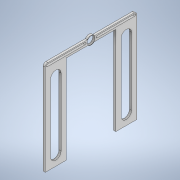
# Autodesk Inventor part: Monitor Part ReDes
Saved by Autodesk Inventor 2020.2 (Build 242310000, 310)
## iProperties
Created: 2020-05-07
Part Number: Monitor Part ReDes
Material: Generic
Document SubType Name: Modeling
Designer: Amaan Khalid
Density: 1 g/cm^3
Appearance: Default
Author: Amaan Khalid
Autodesk Inventor part; units mm, degrees
ref_plane "YZ Plane" through (0, 0, 0) normal (1, 0, 0) x (0, 1, 0)
ref_plane "XZ Plane" through (0, 0, 0) normal (0, 1, 0) x (-1, 0, 0)
ref_plane "XY Plane" through (0, 0, 0) normal (0, 0, 1) x (1, 0, 0)
sketch "Sketch1" plane through (0, 0, 0) normal (1, 0, 0) x (0, 1, 0)
  circle A0 centre (30.6474, 53.9552) radius 5.08
  line L0 (33.2311, 49.5813) -> (33.2311, 1.9563)
  line L1 (33.2311, 58.3291) -> (33.2311, 105.9541)
  line L2 (30.0561, 109.1291) -> (27.0711, 109.1291)
  arc A1 (33.2311, 105.9541) -> (30.0561, 109.1291) centre (30.0561, 105.9541) ccw
  line L3 (30.0561, -1.2187) -> (27.0711, -1.2187)
  arc A2 (30.0561, -1.2187) -> (33.2311, 1.9563) centre (30.0561, 1.9563) ccw
  line L4 (27.0711, 109.1291) -> (27.0711, 57.5631)
  line L5 (27.0711, -1.2187) -> (27.0711, 50.3474)
  line L6 (27.0711, 109.1291) -> (27.0711, 83.7291)
  line L7 (27.0711, 109.1291) -> (-79.6089, 109.1291)
  line L8 (-79.6089, 109.1291) -> (-79.6089, 83.7291)
  line L9 (-79.6089, 83.7291) -> (27.0711, 83.7291)
  line L10 (27.0711, -1.2187) -> (-79.6089, -1.2187)
  line L11 (-79.6089, -1.2187) -> (-79.6089, 24.1813)
  line L12 (27.0711, -1.2187) -> (27.0711, 24.1813)
  line L13 (27.0711, 24.1813) -> (-79.6089, 24.1813)
  circle A3 centre (30.6474, 53.9552) radius 4.7025
  point P0 (33.2311, -1.2187)
  point P1 (33.2311, 109.1291)
  dimension "d3" = 50.8
  dimension "d4" = 50.8
  dimension "d5" = 6.16
  dimension "d6" = 3.175
  dimension "d7" = 3.175
  dimension "d8" = 25.4
  dimension "d9" = 106.68
  dimension "d10" = 106.68
  dimension "d11" = 25.4
  dimension "d13" = 25.4
  constraints: 28 end point, 8 point on circle, 6 point on line, 4 centre point, 4 horizontal, 4 tangent, 3 perpendicular, 3 vertical, 1 coincident
  measures "d3" distance of L0.start point (33.231, -1.219)
  measures "d4" distance of L1.start point (33.231, 109.129)
  measures "d5" distance of point (33.231, 109.129) L2.end
  measures "d6" radius of A1
  measures "d7" radius of A2
  measures "d8" distance of L2.end L6.end
  measures "d9" distance of L2.end L7.end
  measures "d10" distance of L3.end L10.end
  measures "d11" distance of L10.end L11.end
  measures "d13" distance of L3.end L12.end
extrude "Extrusion1" add sketch "Sketch1" along normal blind 2.54 contours A0 | A0 L4 L2 A1 L1 | L0 A2 L3 L5 A0
sketch "Sketch2" plane through (2.54, 0, 0) normal (1, 0, 0) x (0, 0, -1)
  line L0 (-109.1291, 27.0711) -> (-57.5631, 27.0711) projected
  line L1 (-109.1291, 27.0711) -> (-109.1291, -79.6089)
  line L2 (-109.1291, -79.6089) -> (-83.7291, -79.6089)
  line L3 (-83.7291, -79.6089) -> (-83.7291, 27.0711)
  line L4 (-109.1291, 27.0711) -> (-83.7291, 27.0711)
  line L5 (1.2187, 27.0711) -> (1.2187, 30.0561) projected
  line L6 (1.2187, 27.0711) -> (1.2187, -79.6089)
  line L7 (1.2187, -79.6089) -> (-24.1813, -79.6089)
  line L8 (-24.1813, -79.6089) -> (-24.1813, 27.0711)
  line L9 (-50.3474, 27.0711) -> (1.2187, 27.0711) projected
  point P0 (0, 0)
  dimension "d16" = 106.68
  dimension "d17" = 25.4
  dimension "d18" = 106.68
  dimension "d19" = 25.4
  constraints: 14 end point, 3 perpendicular, 2 point on line, 2 vertical, 1 collinear, 1 horizontal
  measures "d16" distance of L0.start L1.end
  measures "d17" distance of L1.end L2.end
  measures "d18" distance of L5.start L6.end
  measures "d19" distance of L6.end L7.end
extrude "Extrusion2" add sketch "Sketch2" against normal up to surface (2.54 mm away)
sketch "Sketch3" plane through (2.54, 0, 0) normal (1, 0, 0) x (0, 0, -1)
  line L0 (-83.7291, -79.6089) -> (-83.7291, 27.0711) projected
  line L1 (-58.3291, 33.2311) -> (-105.9541, 33.2311) projected
  line L2 (-109.1291, 30.0561) -> (-109.1291, -79.6089) projected
  line L3 (-109.1291, -79.6089) -> (-83.7291, -79.6089) projected
  line L4 (-96.4291, 20.7211) -> (-96.4291, 20.7211)
  line L5 (-90.0791, 14.3711) -> (-90.0791, -66.9089)
  line L6 (-96.4291, -73.2589) -> (-96.4291, -73.2589)
  line L7 (-102.7791, -66.9089) -> (-102.7791, 14.3711)
  arc A0 (-96.4291, 20.7211) -> (-102.7791, 14.3711) centre (-96.4291, 14.3711) ccw
  arc A1 (-90.0791, 14.3711) -> (-96.4291, 20.7211) centre (-96.4291, 14.3711) ccw
  arc A2 (-102.7791, -66.9089) -> (-96.4291, -73.2589) centre (-96.4291, -66.9089) ccw
  arc A3 (-96.4291, -73.2589) -> (-90.0791, -66.9089) centre (-96.4291, -66.9089) ccw
  line L8 (-11.4813, 20.7211) -> (-11.4813, 20.7211)
  line L9 (-17.8313, 14.3711) -> (-17.8313, -66.9089)
  line L10 (-11.4813, -73.2589) -> (-11.4813, -73.2589)
  line L11 (-5.1313, -66.9089) -> (-5.1313, 14.3711)
  line L12 (-24.1813, -79.6089) -> (1.2187, -79.6089) projected
  line L13 (-50.3474, 27.0711) -> (-24.1813, 27.0711) projected
  line L14 (1.2187, -79.6089) -> (1.2187, 30.0561) projected
  line L15 (-24.1813, 27.0711) -> (-24.1813, -79.6089) projected
  arc A4 (-11.4813, 20.7211) -> (-17.8313, 14.3711) centre (-11.4813, 14.3711) ccw
  arc A5 (-5.1313, 14.3711) -> (-11.4813, 20.7211) centre (-11.4813, 14.3711) ccw
  arc A6 (-17.8313, -66.9089) -> (-11.4813, -73.2589) centre (-11.4813, -66.9089) ccw
  arc A7 (-11.4813, -73.2589) -> (-5.1313, -66.9089) centre (-11.4813, -66.9089) ccw
  circle A8 centre (-53.9552, 30.6474) radius 4.7025 projected
  line L16 (-58.6577, 30.6474) -> (-61.1977, 30.6474)
  arc A9 (-61.1977, 29.3774) -> (-61.1977, 31.9174) centre (-61.1977, 30.6474) ccw
  line L17 (-109.1291, 30.6474) -> (-106.5891, 30.6474)
  arc A10 (-106.5891, 31.9174) -> (-106.5891, 29.3774) centre (-106.5891, 30.6474) ccw
  line L18 (-106.5891, 31.9174) -> (-61.1977, 31.9174)
  line L19 (-106.5891, 29.3774) -> (-61.1977, 29.3774)
  line L20 (-49.2527, 30.6474) -> (-46.7127, 30.6474)
  arc A11 (-46.7127, 31.9174) -> (-46.7127, 29.3774) centre (-46.7127, 30.6474) ccw
  arc A12 (-1.3213, 29.3774) -> (-1.3213, 31.9174) centre (-1.3213, 30.6474) ccw
  line L21 (-1.3213, 31.9174) -> (-46.7127, 31.9174)
  line L22 (-46.7127, 29.3774) -> (-1.3213, 29.3774)
  point P0 (0, 0)
  dimension "d26" = 6.35
  dimension "d27" = 6.35
  dimension "d28" = 6.35
  dimension "d29" = 6.35
  dimension "d30" = 6.35
  dimension "d31" = 6.35
  dimension "d32" = 6.35
  dimension "d33" = 6.35
  dimension "d34" = 6.35
  dimension "d35" = 6.35
  dimension "d36" = 2.54
  dimension "d37" = 2.54
  dimension "d38" = 2.54
  dimension "d39" = 2.54
  dimension "d40" = 2.54
  dimension "d41" = 2.54
  dimension "d43" = 2.54
  constraints: 30 end point, 26 point on circle, 21 tangent, 12 centre point, 6 equal radius, 5 horizontal, 4 parallel, 3 coincident, 2 perpendicular
  measures "d26" distance from line of L0.end L4
  measures "d27" distance between parallel lines of L0 L5
  measures "d28" distance between parallel lines of L3 L6
  measures "d29" distance between parallel lines of L2 L7
  measures "d30" radius of A0
  measures "d31" distance between parallel lines of L12 L10
  measures "d32" distance between parallel lines of L13 L8
  measures "d33" distance between parallel lines of L14 L11
  measures "d34" distance between parallel lines of L15 L9
  measures "d35" radius of A4
  measures "d36" distance of L16.start L16.end
  measures "d37" diameter of A9
  measures "d38" distance of L17.start L17.end
  measures "d39" diameter of A10
  measures "d40" distance of L20.start L20.end
  measures "d41" diameter of A11
  measures "d43" diameter of A12
extrude "Extrusion3" cut sketch "Sketch3" against normal through all contours L5 A3 A2 L7 A0 A1 | A4 A5 L11 A7 A6 L9 | L19 A10 L18 A9 | L21 A12 L22 A11
body "Solid1"
